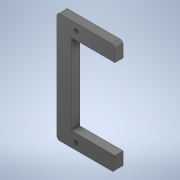
# Autodesk Inventor part: s-10-5_Holder
Saved by Autodesk Inventor 2020 (Build 240168000, 168)
## iProperties
Created: 2020-08-08
Part Number: s-10-5_Holder
Material: Типовые
Document SubType Name: Modeling
Designer: Михаил
Density: 1 g/cm^3
Appearance: По умолчанию
Author: Михаил
Autodesk Inventor part; units mm, degrees
ref_plane "YZ Plane" through (0, 0, 0) normal (1, 0, 0) x (0, 1, 0)
ref_plane "XZ Plane" through (0, 0, 0) normal (0, 1, 0) x (-1, 0, 0)
ref_plane "XY Plane" through (0, 0, 0) normal (0, 0, 1) x (1, 0, 0)
sketch "Эскиз1" plane through (0, 0, 0) normal (0, 0, 1) x (1, 0, 0)
  line L0 (0, 0) -> (39, 0)
  line L1 (39, 0) -> (39, 74)
  line L2 (39, 74) -> (0, 74)
  line L3 (0, 74) -> (0, 0)
  dimension "d0" = 39
  dimension "d1" = 74
  constraints: 8 end point, 2 parallel, 1 horizontal, 1 perpendicular
  measures "d0" distance of L2.end L1.end
  measures "d1" distance of L0.end L1.end
extrude "Выдавливание1" add sketch "Эскиз1" along normal blind 5.5
sketch "Эскиз2" plane through (0, 0, 5.5) normal (0, 0, 1) x (1, 0, 0)
  line L0 (39, 0) -> (39, 74) projected
  line L1 (39, 10) -> (10, 10)
  line L2 (10, 10) -> (10, 64)
  line L3 (10, 64) -> (39, 64)
  line L4 (39, 64) -> (39, 10)
  line L5 (0, 0) -> (39, 0) projected
  line L6 (39, 74) -> (0, 74) projected
  point P0 (39, 64)
  dimension "d4" = 10
  dimension "d5" = 10
  dimension "d6" = 29
  constraints: 8 end point, 2 parallel, 1 horizontal, 1 perpendicular, 1 point on line
  measures "d4" distance between parallel lines of L5 L1
  measures "d5" distance between parallel lines of L6 L3
  measures "d6" distance between parallel lines of L0 L2
extrude "Выдавливание2" cut sketch "Эскиз2" against normal blind 13.5
sketch "Эскиз3" plane through (0, 0, 5.5) normal (0, 0, 1) x (1, 0, 0)
  circle A0 centre (13, 4.5) radius 1.25
  circle A1 centre (13, 69.5) radius 1.25
  line L0 (39, 0) -> (39, 10) projected
  line L1 (39, 64) -> (39, 74) projected
  line L2 (0, 0) -> (39, 0) projected
  line L3 (39, 74) -> (0, 74) projected
  dimension "d9" = 26
  dimension "d10" = 26
  dimension "d11" = 2.5
  dimension "d12" = 2.5
  dimension "d13" = 65
  dimension "d14" = 4.5
  dimension "d15" = 4.5
  constraints: 2 centre point
  measures "d9" distance from line of L0 A0.centre
  measures "d10" distance from line of L1 A1.centre
  measures "d11" diameter of A0
  measures "d12" diameter of A1
  measures "d13" distance of A1.centre A0.centre
  measures "d14" distance from line of L2 A0.centre
  measures "d15" distance from line of L3 A1.centre
extrude "Выдавливание3" cut sketch "Эскиз3" against normal blind 4.5
fillet "Сопряжение1" radius 2 4 edges at (39, 0, 2.75) (39, 74, 2.75) (0, 0, 2.75) (0, 74, 2.75)
